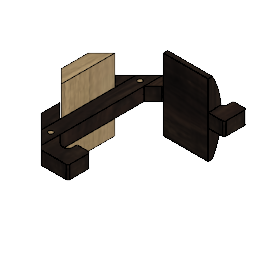
FrenchCleatHeadphoneHook v23 (Autodesk Fusion 360 design; units mm, degrees)
Autodesk Fusion 360 part; units mm, degrees
note: some values were not read from the file. Set by a fixed rule: which sketch regions a step uses.
sketch "Sketch1" plane through (0, 0, 0) normal (0, 0, 1) x (1, 0, 0)
  line L0 (0, 0) -> (0, 76.2)
  line L1 (0, 76.2) -> (-19.05, 57.15)
  line L2 (-19.05, 57.15) -> (-19.05, 19.05)
  line L3 (-19.05, 19.05) -> (0, 0)
  line L4 (0.7937, -1.9163) -> (0.7938, 78.1163)
  line L5 (0.7938, 78.1163) -> (-19.8438, 57.4788)
  line L6 (-19.8438, 57.4788) -> (-19.8438, 18.7212)
  line L7 (-19.8438, 18.7212) -> (0.7937, -1.9163)
  line L8 (-19.8438, 57.4788) -> (-19.8438, 84.4196)
  line L9 (-19.8438, 84.4196) -> (24.3136, 128.5769)
  line L10 (32.2044, 109.5269) -> (0.7938, 78.1163)
  line L11 (19.8438, 97.1663) -> (19.8438, -47.9071)
  line L12 (19.8438, 97.1663) -> (19.8438, 124.1071)
  line L13 (0.7938, 78.1163) -> (0.7937, 105.0571)
  line L14 (0.7937, -1.9163) -> (29.9725, -31.095)
  line L15 (-19.8438, 18.7212) -> (-19.8438, -8.2196)
  line L16 (-19.8438, -8.2196) -> (24.3136, -52.3769)
  line L17 (0.7937, -1.9163) -> (0.7937, -28.8571)
  line L18 (26.1096, -53.1208) -> (60.6175, -53.1208)
  line L19 (63.1575, -50.5808) -> (63.1575, -23.9108)
  line L20 (60.6175, -21.3708) -> (46.6475, -21.3708)
  line L21 (44.1075, -23.9108) -> (44.1075, -27.7208)
  line L22 (37.7575, -34.0708) -> (37.1567, -34.0708)
  arc A0 (37.7575, -34.0708) -> (44.1075, -27.7208) centre (37.7575, -27.7208) ccw
  arc A1 (29.9725, -31.095) -> (37.1567, -34.0708) centre (37.1567, -23.9108) ccw
  arc A2 (46.6475, -21.3708) -> (44.1075, -23.9108) centre (46.6475, -23.9108) ccw
  arc A3 (63.1575, -23.9108) -> (60.6175, -21.3708) centre (60.6175, -23.9108) ccw
  arc A4 (60.6175, -53.1208) -> (63.1575, -50.5808) centre (60.6175, -50.5808) ccw
  arc A5 (24.3136, -52.3769) -> (26.1096, -53.1208) centre (26.1096, -50.5808) ccw
  line L23 (26.1096, 129.3208) -> (98.0825, 129.3208)
  line L24 (101.2575, 132.4958) -> (101.2575, 139.4808)
  line L25 (103.7975, 142.0208) -> (117.7675, 142.0208)
  line L26 (120.3075, 139.4808) -> (120.3075, 112.8108)
  line L27 (117.7675, 110.2708) -> (34.0004, 110.2708)
  arc A6 (34.0004, 110.2708) -> (32.2044, 109.5269) centre (34.0004, 107.7308) ccw
  arc A7 (26.1096, 129.3208) -> (24.3136, 128.5769) centre (26.1096, 126.7808) ccw
  arc A8 (98.0825, 129.3208) -> (101.2575, 132.4958) centre (98.0825, 132.4958) ccw
  arc A9 (103.7975, 142.0208) -> (101.2575, 139.4808) centre (103.7975, 139.4808) ccw
  arc A10 (120.3075, 139.4808) -> (117.7675, 142.0208) centre (117.7675, 139.4808) ccw
  arc A11 (117.7675, 110.2708) -> (120.3075, 112.8108) centre (117.7675, 112.8108) ccw
  line L28 (0.7937, 105.0571) -> (19.8438, 97.1663) construction
  line L29 (19.8438, 124.1071) -> (0.7938, 78.1163) construction
  circle A12 centre (10.3188, 101.1117) radius 3.175
  line L30 (0.7937, -1.9163) -> (19.8438, -47.9071) construction
  line L31 (19.8438, -20.9663) -> (0.7937, -28.8571) construction
  circle A13 centre (10.3187, -24.9117) radius 3.175
  dimension "d1" = 76.2
  dimension "d2" = 45
  dimension "d3" = 45
  dimension "d4" = 19.05
  dimension "d5" = 0.7937
  dimension "d6" = 19.05
  dimension "d8" = 19.05
  dimension "d9" = 19.05
  dimension "d10" = 63.5
  dimension "d11" = 38.1
  dimension "d12" = 31.75
  dimension "d13" = 19.05
  dimension "d14" = 19.05
  dimension "d15" = 6.35
  dimension "d16" = 10.16
  dimension "d17" = 2.54
  dimension "d18" = 2.54
  dimension "d19" = 2.54
  dimension "d20" = 2.54
  dimension "d23" = 19.05
  dimension "d24" = 19.05
  dimension "d25" = 12.7
  dimension "d26" = 76.2
  dimension "d27" = 2.54
  dimension "d28" = 2.54
  dimension "d29" = 3.175
  dimension "d30" = 2.54
  dimension "d31" = 2.54
  dimension "d46" = 6.35
  dimension "d47" = 6.35
  measures "d1" distance of L0.start
  measures "d2" angle of L0 L1
  measures "d3" angle of L0 L3
  measures "d4" distance of L0 L2
  measures "d5" distance of L0
  measures "d6" distance of L9 L10
  measures "d8" distance of L4 L11
  measures "d9" distance of L14 L16
  measures "d10" distance of L0.start
  measures "d14" distance of L18 L22
  measures "d15" radius of A0
  measures "d16" radius of A1
  measures "d19" radius of A4
  measures "d20" radius of A5
  measures "d24" distance of L23 L27
  measures "d27" radius of A6
  measures "d28" radius of A7
  measures "d29" radius of A8
  measures "d30" radius of A9
  measures "d31" radius of A11
  measures "d46" diameter of A12
  measures "d47" diameter of A13
extrude "Extrude1" add sketch "Sketch1" against normal blind 9.525 contours L9 L10 L12 L13 | L5 L8 L9 L13 | L9 L10 L12 L23 L24 L25 L26 L27 A6 A7 A8 A9 A10 A11 | A12 makes body 1 in component "Component"
extrude "Extrude2" add sketch "Sketch1" along normal blind 9.525 contours L5 L8 L9 L13 | L9 L10 L12 L23 L24 L25 L26 L27 A6 A7 A8 A9 A10 A11 bodies 1 in component "Component"
extrude "Extrude1'" add sketch "Sketch1" along normal blind 9.525 separate body contours L4 L10 L11 L14 | L11 L14 L16 L17 | L9 L10 L12 L13 | A12 | A13 makes body 2 in component "Component'"
extrude "Extrude2'" add sketch "Sketch1" against normal blind 9.525 contours L4 L10 L11 L14 bodies 2 in component "Component'"
extrude "Extrude1''" add sketch "Sketch1" against normal blind 9.525 separate body contours L7 L15 L16 L17 | L11 L14 L16 L17 | L11 L14 L16 L18 L19 L20 L21 L22 A0 A1 A2 A3 A4 A5 | A13 makes body 3 in component "Component''"
extrude "Extrude2''" add sketch "Sketch1" along normal blind 9.525 contours L7 L15 L16 L17 | L11 L14 L16 L18 L19 L20 L21 L22 A0 A1 A2 A3 A4 A5 bodies 3 in component "Component''"
extrude "Extrude1'''" add sketch "Sketch1" along normal mid plane 101.6 separate body contours L0 L1 L2 L3 makes body 4 in component "Component'''"
extrude "Extrude3" cut sketch "Sketch1" against normal through all contours A12 bodies 1 in component "Component"
extrude "Extrude3'" cut sketch "Sketch1" along normal through all contours A12 bodies 2 in component "Component'"
extrude "Extrude4" cut sketch "Sketch1" along normal through all contours A13 bodies 2 in component "Component'"
extrude "Extrude3''" cut sketch "Sketch1" against normal through all contours A13 bodies 3 in component "Component''"
extrude "Extrude1''''" add sketch "Sketch1" along normal mid plane 19.05 separate body contours A12 makes body 5 in component "Component''''"
extrude "Extrude1'''''" add sketch "Sketch1" along normal blind 9.525 and the other way blind 0 separate body contours A13 makes body 6 in component "Component'''''"
extrude "Extrude2'''" add sketch "Sketch1" against normal blind 9.525 contours A13 bodies 6 in component "Component'''''"
ref_plane "WorkPlane1" through (101.2575, 126.1458, 0) normal (1, 0, 0) x (0, -1, 0)
sketch "Sketch2" plane through (101.2575, 126.1458, 0) normal (1, 0, 0) x (0, 1, 0)
  line L0 (-16.6189, -9.525) -> (-16.6189, 9.525)
  line L1 (-15.875, 0) -> (-15.875, 50.8)
  line L2 (-15.875, 50.8) -> (-9.525, 50.8)
  line L3 (-15.875, 0) -> (-15.875, -50.8)
  line L4 (-15.875, -50.8) -> (-9.525, -50.8)
  line L5 (-15.875, 0) -> (3.175, 0)
  arc A0 (-9.525, -50.8) -> (-9.525, 50.8) centre (-104.775, 0) ccw
  dimension "d61" = 50.8
  dimension "d62" = 6.35
  dimension "d63" = 90
  dimension "d64" = 50.8
  dimension "d65" = 6.35
  dimension "d66" = 19.05
  measures "d63" angle of L1 L2
extrude "Extrude1''''''" add sketch "Sketch2" against normal blind 73.66 separate body makes body 7 in component "Component''''''"
ref_plane "WorkPlane2" through (64.4275, 129.3208, 0) normal (0, -1, 0) x (0, 0, 1)
ref_plane "WorkPlane1" through (64.4275, 129.3208, 0) normal (0, -1, 0) x (0, 0, 1) in component "Component''''''"
sketch "Sketch1 (2)" plane through (63.1575, 129.3208, 0) normal (0, -1, 0) x (1, 0, 0) in component "Component''''''"
  line L0 (38.1, 9.779) -> (-38.0387, 9.779)
  line L1 (-30.9532, -9.525) -> (-83.0013, -9.525)
  line L2 (38.1, -50.8) -> (38.1, 50.8)
  line L3 (-38.0387, -9.525) -> (38.1, -9.525)
  line L4 (38.1, 9.525) -> (38.1, -9.525)
  line L5 (-38.0387, -9.525) -> (-38.0387, 9.779)
  line L6 (-38.0387, 0.127) -> (38.1, 0)
  dimension "d79" = 19.304
  measures "d79" distance of L0 L3
extrude "Extrude2''''" cut sketch "Sketch1 (2)" along normal blind 9.525 bodies 7 in component "Component''''''"
move_face "OffsetFaces1" offset -3.81 1 faces at (101.2575, 113.4458, -3.175) on bodies 7 in component "Component''''''"
extrude "Extrude3'''" cut 1 faces at (27.5975, 113.4458, -3.175) along direction (1, 0, 0) blind 6.35 on bodies 7 bodies 7 in component "Component''''''"
sketch "Sketch1 (3)" plane through (0, 0, 9.525) normal (0, 0, 1) x (-1, 0, 0) in component "Component"
  line L0 (-34.0004, -110.2708) -> (-117.7675, -110.2708)
  arc A0 (-117.7675, -110.2708) -> (-120.3075, -112.8108) centre (-117.7675, -112.8108) ccw
  line L1 (-120.3075, -112.8108) -> (-120.3075, -139.4808)
  arc A1 (-120.3075, -139.4808) -> (-117.7675, -142.0208) centre (-117.7675, -139.4808) ccw
  line L2 (-117.7675, -142.0208) -> (-103.7975, -142.0208)
  arc A2 (-103.7975, -142.0208) -> (-101.2575, -139.4808) centre (-103.7975, -139.4808) ccw
  line L3 (-101.2575, -139.4808) -> (-101.2575, -132.4958)
  arc A3 (-98.0825, -129.3208) -> (-101.2575, -132.4958) centre (-98.0825, -132.4958) ccw
  line L4 (-98.0825, -129.3208) -> (-26.1096, -129.3208)
  arc A4 (-26.1096, -129.3208) -> (-24.3136, -128.5769) centre (-26.1096, -126.7808) ccw
  line L5 (-24.3136, -128.5769) -> (-19.8438, -124.1071)
  line L6 (-19.8438, -124.1071) -> (-19.8438, -97.1663)
  line L7 (-19.8438, -97.1663) -> (-32.2044, -109.5269)
  arc A5 (-34.0004, -110.2708) -> (-32.2044, -109.5269) centre (-34.0004, -107.7308) ccw
  line L8 (-34.0004, -110.2708) -> (-33.9475, -119.9228)
  line L9 (-33.9475, -119.9228) -> (-97.7015, -119.9228)
  line L10 (-97.7015, -119.9228) -> (-97.7015, -110.2708)
  dimension "d77" = 63.754
  dimension "d78" = 9.652
extrude "Extrude4'" cut sketch "Sketch1 (3)" against normal through all contours L0 L8 L9 L10 bodies 1 in component "Component"
component "Component" placed x (1, 0, 0) y (0, 1, 0) z (0, 0, 1) at (0, 0, 0)
component "Component'" placed x (1, 0, 0) y (0, 1, 0) z (0, 0, 1) at (0, 0, 0)
component "Component''" placed x (1, 0, 0) y (0, 1, 0) z (0, 0, 1) at (-0.0928, -0.2644, -0.0528)
component "Component'''" placed x (1, 0, 0) y (0, 1, 0) z (0, 0, 1) at (0, 0, 0)
component "Component''''" placed x (1, 0, 0) y (0, 1, 0) z (0, 0, 1) at (0, 0, 0)
component "Component'''''" placed x (1, 0, 0) y (0, 1, 0) z (0, 0, 1) at (0, 0, 0)
component "Component''''''" placed x (1, 0, 0) y (0, 1, 0) z (0, 0, 1) at (0, 0, 0)
